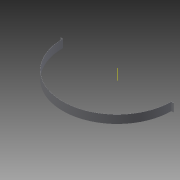
# Autodesk Inventor part: Band
Saved by Autodesk Inventor 2015 (Build 190159000, 159)
## iProperties
Created: 2014-06-19
Part Number: Band
Material: Generic
Document SubType Name: Modeling
Designer: Aki
Density: 1 g/cm^3
Appearance: Default
Author: Aki
Autodesk Inventor part; units mm, degrees
ref_plane "YZ Plane" through (0, 0, 0) normal (1, 0, 0) x (0, 1, 0)
ref_plane "XY Plane" through (0, 0, 0) normal (0, 0, 1) x (1, 0, 0)
sketch "Sketch1" plane through (0, 0, 0) normal (0, 1, 0) x (-1, 0, 0)
  arc A0 (401, 0) -> (-401, 0) centre (0, 0) ccw
  line L0 (0, 0) -> (-401, 0) construction
  line L1 (0, 0) -> (401, 0) construction
  arc A1 (402, 0) -> (-402, 0) centre (0, 0) ccw
  line L2 (0, 0) -> (-402, 0) construction
  line L3 (0, 0) -> (402, 0) construction
  line L4 (402, 0) -> (401, 0)
  line L5 (-402, 0) -> (-401, 0)
  dimension "d0" = 401
  dimension "d1" = 180
  dimension "d2" = 402
  dimension "d3" = 180
  constraints: 12 end point, 4 point on circle, 2 centre point, 2 coincident, 1 collinear
  measures "d0" radius of A0
  measures "d1" angle of L0 L1
  measures "d2" radius of A1
  measures "d3" angle of L2 L3
extrude "Extrusion1" add sketch "Sketch1" along normal blind 60
sketch "Sketch2" plane through (0, 0, 0) normal (0, 1, 0) x (-1, 0, 0)
  line L0 (-402, 0) -> (-417, 0)
  line L1 (-417, 0) -> (-417, 2)
  line L2 (-417, 2) -> (-402, 2)
  line L3 (-402, 2) -> (-402, 0)
  point P0 (0, 0)
  dimension "d6" = 15
  dimension "d7" = 2
  constraints: 8 end point, 2 parallel, 1 horizontal, 1 perpendicular
  measures "d6" distance of L1.end L2.end
  measures "d7" distance of L0.end L1.end
extrude "Extrusion2" add sketch "Sketch2" along normal blind 60
sketch "Sketch3" plane through (0, 0, 0) normal (0, 1, 0) x (-1, 0, 0)
  line L0 (402, 0) -> (417, 0)
  line L1 (417, 0) -> (417, 2)
  line L2 (417, 2) -> (402, 2)
  line L3 (402, 2) -> (402, 0)
  point P0 (0, 0)
  dimension "d10" = 15
  dimension "d11" = 2
  constraints: 8 end point, 2 parallel, 1 horizontal, 1 perpendicular
  measures "d10" distance of L2.end L1.end
  measures "d11" distance of L1.end L0.end
extrude "Extrusion3" add sketch "Sketch3" along normal blind 60
ref_plane "Work Plane1" through (0, 30, 0) normal (0, 1, 0) x (-1, 0, 0)
body "Solid1"
